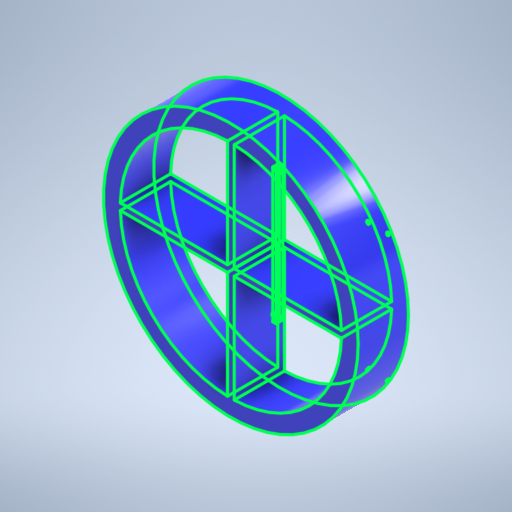
# Autodesk Inventor part: SUJETADOR_MICRO
Saved by Autodesk Inventor 2025 (Build 290162000, 162)
## iProperties
Created: 2024-07-26
Part Number: SUJETADOR_MICRO
Material: Generic
Document SubType Name: Modeling
Designer: Richard
Density: 1 g/cm^3
Appearance: Default
Author: Richard
Autodesk Inventor part; units mm, degrees
ref_plane "YZ Plane" through (0, 0, 0) normal (1, 0, 0) x (0, 1, 0)
ref_plane "XZ Plane" through (0, 0, 0) normal (0, 1, 0) x (-1, 0, 0)
ref_plane "XY Plane" through (0, 0, 0) normal (0, 0, 1) x (1, 0, 0)
sketch "Sketch1" plane through (0, 0, 0) normal (0, 0, 1) x (1, 0, 0)
  circle A0 centre (0, 0) radius 38
  circle A1 centre (0, 0) radius 33
  dimension "d0" = 76
  dimension "d1" = 66
  constraints: 2 centre point, 2 coincident
  measures "d0" diameter of A0
  measures "d1" diameter of A1
extrude "Extrusion1" add sketch "Sketch1" along normal blind 15
sketch "Sketch2" plane through (0, 0, 0) normal (0, 0, -1) x (-1, 0, 0)
  circle A0 centre (0, 0) radius 33 projected
  line L0 (0.0152, 1) -> (-32.9848, 1)
  line L1 (0.0152, -1) -> (-32.9848, -1)
  line L2 (0.0152, 1) -> (-12.0152, 1)
  circle A1 centre (0, 0) radius 33
  line L3 (0.0152, -1) -> (0.0152, 1)
  line L4 (-1, 0.0152) -> (-1, -32.9848)
  line L5 (1, 0.0152) -> (1, -32.9848)
  line L6 (-0.0152, -1) -> (32.9848, -1)
  line L7 (-0.0152, 1) -> (32.9848, 1)
  line L8 (1, -0.0152) -> (1, 32.9848)
  line L9 (-1, -0.0152) -> (-1, 32.9848)
  point P0 (-1, 1)
  point P1 (-1, -1)
  point P2 (1, -1)
  point P3 (1, 1)
  dimension "d12" = 2
  dimension "d17" = 66
  dimension "d18" = 33
  dimension "d19" = 33
  dimension "d22" = 360
  constraints: 20 end point, 2 point on circle, 1 centre point, 1 coincident, 1 parallel, 1 vertical, 25 other
  measures "d12" distance of L0.start L1.start
  measures "d17" diameter of A1
  measures "d18" distance of L0.start L0.end
  measures "d19" distance of L1.start L1.end
extrude "Extrusion2" add sketch "Sketch2" against normal blind 15 contours A0 L6 L5 L8 L7 | L8 L7 L0 L9 A0 | L8 L5 L6 L3 L7 | A0 L4 L1 L6 L5 | L3 L1 L4 L9 L0 | L0 L9 L4 L1 A0
sketch "Sketch3" plane through (0, 0, 0) normal (0, 0, -1) x (-1, 0, 0)
  line L0 (0, 20) -> (-0.5, 20)
  line L1 (-0.5, 20) -> (-0.5, -20)
  line L2 (-0.5, -20) -> (0.5, -20)
  line L3 (0.5, -20) -> (0.5, 20)
  line L4 (0.5, 20) -> (0, 20)
  point P0 (0, 0)
  dimension "d27" = 20
  dimension "d29" = 40
  dimension "d30" = 1
  dimension "d31" = 40
  constraints: 10 end point, 2 perpendicular, 1 horizontal, 1 point on line
  measures "d27" distance of point (0, 0) L0.start
  measures "d29" distance of L0.end L1.end
  measures "d30" distance of L1.end L2.end
  measures "d31" distance of L2.end L3.end
extrude "Extrusion3" cut sketch "Sketch3" against normal blind 2
sketch "Sketch4" plane through (-1, 1, 0) normal (-1, 0, 0) x (0, 0, 1)
  point P0 (0, -1)
  point P1 (1.0253, 17.9677)
hole "Hole1" at (-1, 18.9677, 1.0253) direction (1, 0, 0) diameter 0.7 end through all
sketch "Sketch5" plane through (-1, -32.9848, 0) normal (-1, 0, 0) x (0, 0, 1)
  point P0 (0, 32.9848)
  point P1 (1.4149, 14.4794)
hole "Hole2" at (-1, -18.5055, 1.4149) direction (1, 0, 0) diameter 0.7 end through all
body "Solid1"
